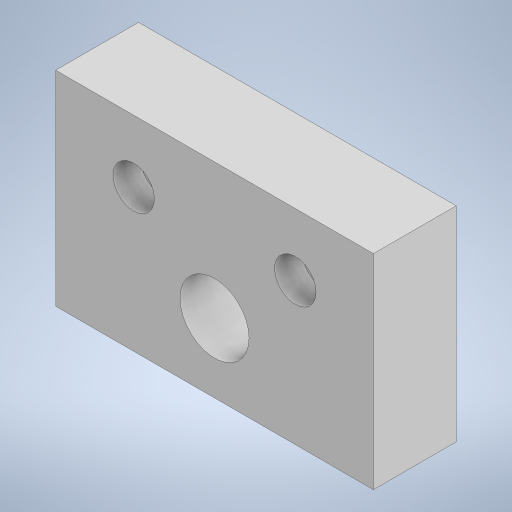
# Autodesk Inventor part: cam m6 replacement v01
Saved by Autodesk Inventor 2023 (Build 270158000, 158)
## iProperties
Created: 2024-07-08
Part Number: cam m6 replacement v01
Material: Generic
Document SubType Name: Modeling
Designer: Akramilab
Density: 1 g/cm^3
Appearance: Default
Author: Akramilab
Autodesk Inventor part; units mm, degrees
ref_plane "YZ Plane" through (0, 0, 0) normal (1, 0, 0) x (0, 1, 0)
ref_plane "XZ Plane" through (0, 0, 0) normal (0, 1, 0) x (-1, 0, 0)
ref_plane "XY Plane" through (0, 0, 0) normal (0, 0, 1) x (1, 0, 0)
sketch "Sketch1" plane through (0, 0, 0) normal (0, 0, 1) x (1, 0, 0)
  line L0 (0, 0) -> (23, 0)
  line L1 (23, 0) -> (23, -14.8)
  line L2 (23, -14.8) -> (0, -14.8)
  line L3 (0, -14.8) -> (0, 0)
  circle A0 centre (5.65, -4.5) radius 1.5
  circle A1 centre (17.35, -4.5) radius 1.5
  circle A2 centre (11.5, -9.8) radius 2.5
  dimension "d0" = 23
  dimension "d1" = 14.8
  dimension "d2" = 4.5
  dimension "d3" = 11.7
  dimension "d4" = 5.65
  dimension "d5" = 5.65
  dimension "d6" = 11.5
  dimension "d7" = 5
  dimension "d8" = 3
  dimension "d9" = 3
  dimension "d10" = 5
  constraints: 8 end point, 3 centre point, 3 coincident, 2 parallel, 1 horizontal, 1 perpendicular
  measures "d0" distance of L1.end L2.end
  measures "d1" distance of L0.end L1.end
  measures "d2" distance from line of point (5.65, -4.5) L0
  measures "d3" distance of point (17.35, -4.5) point (5.65, -4.5)
  measures "d4" distance from line of point (5.65, -4.5) L3
  measures "d5" distance from line of L1 point (17.35, -4.5)
  measures "d6" distance from line of L3 point (11.5, -9.8)
  measures "d7" distance from line of L2 point (11.5, -9.8)
  measures "d8" diameter of A0
  measures "d9" diameter of A1
  measures "d10" diameter of A2
extrude "Extrusion1" add sketch "Sketch1" along normal blind 6
sketch "Sketch2" plane through (0, 0, 0) normal (0, 0, -1) x (-1, 0, 0)
  circle A0 centre (-17.35, -4.5) radius 1.5 projected
  circle A1 centre (-17.35, -4.5) radius 2.5
  circle A2 centre (-5.65, -4.5) radius 1.5 projected
  circle A3 centre (-5.65, -4.5) radius 2.5
  point P0 (0, 0)
  dimension "d13" = 5
  dimension "d14" = 5
  constraints: 2 centre point, 2 coincident
  measures "d13" diameter of A1
  measures "d14" diameter of A3
extrude "Extrusion2" cut sketch "Sketch2" against normal blind 4
equation "\"d4\" = -0.5 * d3 + 0.5 * d0"
equation "\"d5\" = d4"
equation "\"d6\" = 0.5 * d0"
equation "\"d9\" = d8"
equation "\"d14\" = d13"
body "Solid1"
